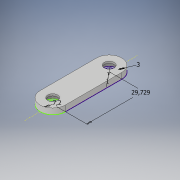
# Autodesk Inventor part: BeltDriveTestHolder
Saved by Autodesk Inventor 2018.3 (Build 223284000, 284)
## iProperties
Created: 2018-07-29
Part Number: BeltDriveTestHolder
Material: Generisch
Document SubType Name: Modeling
Designer: JochenAlt
Density: 1 g/cm^3
Appearance: Vorgabe
Author: JochenAlt
Autodesk Inventor part; units mm, degrees
ref_plane "YZ Plane" through (0, 0, 0) normal (1, 0, 0) x (0, 1, 0)
ref_plane "XZ Plane" through (0, 0, 0) normal (0, 1, 0) x (-1, 0, 0)
ref_plane "XY Plane" through (0, 0, 0) normal (0, 0, 1) x (1, 0, 0)
sketch "Skizze1" plane through (0, 0, 0) normal (0, 0, 1) x (1, 0, 0)
  circle A0 centre (0, 0) radius 3.6
  line L0 (0, 44.9148) -> (0, -15.1858) construction
  line L1 (-9.24, 0) -> (9.24, 0) construction
  circle A1 centre (0, 29.729) radius 3.6
  line L2 (0, 29.729) -> (0, 0) construction
  line L3 (6.6, 29.729) -> (6.6, 0)
  line L4 (-6.6, 0) -> (-6.6, 29.729)
  arc A2 (6.6, 29.729) -> (-6.6, 29.729) centre (0, 29.729) ccw
  arc A3 (-6.6, 0) -> (6.6, 0) centre (0, 0) ccw
  circle A4 centre (0, 29.729) radius 2.6
  circle A5 centre (0, 0) radius 2.6
  point P0 (0, 14.8645)
  dimension "d1" = 7.2
  dimension "d2" = 29.729
  dimension "d3" = 1
  dimension "d4" = 3
  constraints: 8 end point, 6 centre point, 4 point on circle, 4 tangent, 2 coincident, 2 equal radius, 1 midpoint, 1 parallel, 1 perpendicular, 1 point on line
  measures "d1" diameter of A0
  measures "d2" distance of L2.start point (0, 0)
  measures "d3" radial gap between concentric circles of A1 A4
  measures "d4" radial gap between concentric circles of A1 A2
extrude "Extrusion1" add sketch "Skizze1" along normal blind 2 contours L3 A3 L4 A2
extrude "Extrusion2" add sketch "Skizze1" along normal blind 1 from surface at 2 contours A0 | A1 | L3 A3 L4 A2
